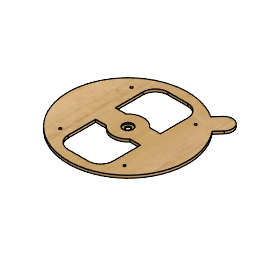
LB1-LB9 - Leveling Base Subassembly (Autodesk Fusion 360 archive; units mm, degrees)
design "LB3 - Bucket Adapter"
Autodesk Fusion 360 part; units mm, degrees
sketch "Sketch1" plane through (0, 0, 0) normal (0, 0, 1) x (1, 0, 0)
  circle A0 centre (-64.5, 71.5) radius 2.25
  circle A1 centre (64.5, 71.5) radius 2.25
  circle A2 centre (-64.5, -71.5) radius 2.25
  circle A3 centre (64.5, -71.5) radius 2.25
  line L0 (20, 100) -> (-20, 100)
  line L1 (-20, -100) -> (20, -100)
  arc A4 (-20, 100) -> (-45, 75) centre (-20, 75) ccw
  arc A5 (45, 75) -> (20, 100) centre (20, 75) ccw
  arc A6 (20, -100) -> (45, -75) centre (20, -75) ccw
  arc A7 (-45, -75) -> (-20, -100) centre (-20, -75) ccw
  line L2 (45, 20) -> (-45, -20) construction
  circle A8 centre (0, 0) radius 5
  line L3 (64.5, 71.5) -> (-64.5, 71.5) construction
  line L4 (-64.5, 71.5) -> (-64.5, -71.5) construction
  line L5 (-64.5, -71.5) -> (64.5, -71.5) construction
  line L6 (64.5, -71.5) -> (64.5, 71.5) construction
  line L7 (64.5, 71.5) -> (-64.5, -71.5) construction
  line L8 (-64.5, 71.5) -> (64.5, -71.5) construction
  line L9 (45, 20) -> (23.6854, 20)
  line L10 (-23.6854, 20) -> (-45, 20)
  line L11 (-45, 75) -> (-45, 20)
  line L12 (-45, -20) -> (-45, -75)
  arc A9 (-23.6854, -20) -> (23.6854, -20) centre (0, 0) ccw
  arc A10 (23.6854, 20) -> (-23.6854, 20) centre (0, 0) ccw
  line L13 (45, -75) -> (45, -20)
  line L14 (45, 20) -> (45, 75)
  line L15 (-45, 20) -> (4.5691, -2.0307) construction
  line L16 (28.3282, -12.5903) -> (45, -20) construction
  line L17 (-45, -20) -> (-23.6854, -20)
  line L18 (23.6854, -20) -> (45, -20)
  line L19 (91.0962, 100.9826) -> (104.4615, 88.9257) construction
  line L20 (91.0962, 100.9826) -> (77.7308, 113.0394) construction
  line L21 (104.4615, 88.9257) -> (92.8349, 76.0373)
  line L22 (77.7308, 113.0394) -> (66.1042, 100.151)
  arc A11 (104.4615, 88.9257) -> (77.7308, 113.0394) centre (91.0962, 100.9826) ccw
  arc A12 (66.1042, 100.151) -> (92.8349, 76.0373) centre (0, 0) ccw
  dimension "d14" = 4.5
  dimension "d15" = 4.5
  dimension "d16" = 4.5
  dimension "d17" = 4.5
  dimension "d20" = 240
  dimension "d21" = 25
  dimension "d23" = 40
  dimension "d24" = 10
  dimension "d25" = 62
  dimension "d26" = 129
  dimension "d27" = 143
  dimension "d29" = 36
  dimension "d33" = 45
  dimension "d34" = 100
  dimension "d35" = 100
  dimension "d36" = 149.4615
  dimension "d37" = 132.054
  dimension "d38" = 213.0394
  dimension "d39" = 18.2443
  dimension "d40" = 18
  constraint horizontal L0
  constraint perpendicular L0 L11
  constraint parallel L0 L1
  constraint parallel L11 L13
  constraint tangent L0 A4
  constraint tangent A4 L11
  constraint tangent A5 L13
  constraint tangent L0 A5
  constraint equal A4 A5
  constraint tangent L1 A6
  constraint tangent A6 L13
  constraint equal A4 A6
  constraint tangent A7 L11
  constraint tangent L1 A7
  constraint equal A4 A7
  constraint horizontal L9
  constraint parallel L9 L17
  constraint coincident L2 A8.centre
  constraint coincident A8.centre L15
  constraint coincident A8.centre A9.centre
  constraint concentric A8 A12
  constraint horizontal L3
  constraint perpendicular L3 L4
  constraint parallel L3 L5
  constraint parallel L4 L6
  constraint coincident L7 A8.centre
  constraint coincident L8 A8.centre
  constraint collinear L9 L10
  constraint coincident L10.start A9
  constraint coincident L9.end A9
  constraint collinear L11 L12
  constraint coincident L16.start L15
  constraint concentric A9 A10
  constraint collinear L13 L14
  constraint coincident A8 L15.end
  constraint collinear L15 L16
  constraint coincident A9.end L17
  constraint collinear L17 L18
  constraint coincident L19.start L20.start
  constraint tangent L21 A11
  constraint tangent L22 A11
  constraint concentric A8 A9
  constraint coincident A2.centre L4.end
  constraint coincident A1.centre L3.start
  constraint coincident A3.centre L5.end
  constraint coincident A0.centre L3.end
  measures "d14" diameter of A0
  measures "d15" diameter of A1
  measures "d16" diameter of A2
  measures "d17" diameter of A3
  measures "d20" diameter of A12
  measures "d21" radius of A4
  measures "d23" distance of L10.end L2.end
  measures "d24" diameter of A8
  measures "d25" diameter of A9
  measures "d26" distance of A2.centre A3.centre
  measures "d27" distance of A0.centre A2.centre
  measures "d29" diameter of A11
  measures "d33" distance of A8.centre L11
  measures "d34" distance of A8.centre L1
  measures "d35" distance of A8.centre L0
  measures "d36" distance of L11 L19.end
  measures "d37" angle of L3 L21
  measures "d38" distance of L1 L20.end
  measures "d39" distance of L13.end L16.start
  measures "d40" distance of L7 L21
extrude "Extrude1" add sketch "Sketch1" along normal blind 5.2
sketch "Sketch4" plane through (0, 0, 5.2) normal (0, 0, 1) x (-1, 0, 0)
  circle A0 centre (-64.5, 71.5) radius 2.25
  circle A1 centre (64.5, 71.5) radius 2.25
  line L0 (-45, -20) -> (-23.6854, -20)
  arc A2 (-23.6854, -20) -> (23.6854, -20) centre (0, 0) ccw
  line L1 (23.6854, -20) -> (45, -20)
  line L2 (45, -20) -> (45, -75)
  arc A3 (20, -100) -> (45, -75) centre (20, -75) ccw
  line L3 (20, -100) -> (-20, -100)
  arc A4 (-45, -75) -> (-20, -100) centre (-20, -75) ccw
  line L4 (-45, -75) -> (-45, -20)
  circle A5 centre (64.5, -71.5) radius 2.25
  circle A6 centre (0, 0) radius 5
  line L5 (45, 75) -> (45, 20)
  line L6 (45, 20) -> (23.6854, 20)
  arc A7 (23.6854, 20) -> (-23.6854, 20) centre (0, 0) ccw
  line L7 (-23.6854, 20) -> (-45, 20)
  line L8 (-45, 20) -> (-45, 75)
  arc A8 (-20, 100) -> (-45, 75) centre (-20, 75) ccw
  line L9 (-20, 100) -> (20, 100)
  arc A9 (45, 75) -> (20, 100) centre (20, 75) ccw
  circle A10 centre (-64.5, -71.5) radius 2.25
  arc A11 (-104.4615, -88.9257) -> (-77.7308, -113.0394) centre (-91.0962, -100.9826) ccw
  line L10 (-77.7308, -113.0394) -> (-66.1042, -100.151)
  arc A12 (-66.1042, -100.151) -> (-92.8349, -76.0373) centre (0, 0) ccw
  line L11 (-92.8349, -76.0373) -> (-104.4615, -88.9257)
  circle A13 centre (0, 0) radius 10
  dimension "d30" = 20
  constraint concentric A2 A13
  measures "d30" diameter of A13
extrude "Extrude3" cut sketch "Sketch4" against normal blind 2.6 contours A13
equation "d31 = ( -5.2 / 2 ) * 1 mm"

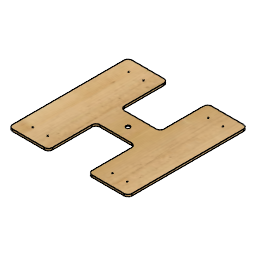
design "LB1 - Baseplate"
Autodesk Fusion 360 part; units mm, degrees
sketch "Sketch1" plane through (0, 0, 0) normal (0, 0, 1) x (1, 0, 0)
  line L0 (40, 31) -> (-40, 31)
  line L1 (-40, -31) -> (40, -31)
  line L2 (50, 31) -> (-50, -31) construction
  line L3 (-50, 31) -> (50, -31) construction
  line L4 (151, 31) -> (151, 141)
  line L5 (141, 151) -> (60, 151)
  line L6 (50, 141) -> (50, 41)
  line L7 (151, -31) -> (151, -141)
  line L8 (141, -151) -> (60, -151)
  line L9 (50, -141) -> (50, -41)
  line L10 (151, -31) -> (151, 31)
  line L11 (0, 0) -> (0, 31) construction
  line L12 (-141, 151) -> (-60, 151)
  line L13 (-50, 141) -> (-50, 41)
  line L14 (-151, 31) -> (-151, 141)
  line L15 (-151, -31) -> (-151, 31)
  line L16 (-141, -151) -> (-60, -151)
  line L17 (-50, -141) -> (-50, -41)
  line L18 (-151, -31) -> (-151, -141)
  circle A0 centre (0, 0) radius 5
  arc A1 (-141, 151) -> (-151, 141) centre (-141, 141) ccw
  arc A2 (-50, 141) -> (-60, 151) centre (-60, 141) ccw
  arc A3 (60, 151) -> (50, 141) centre (60, 141) ccw
  arc A4 (151, 141) -> (141, 151) centre (141, 141) ccw
  arc A5 (-151, -141) -> (-141, -151) centre (-141, -141) ccw
  arc A6 (-60, -151) -> (-50, -141) centre (-60, -141) ccw
  arc A7 (50, -141) -> (60, -151) centre (60, -141) ccw
  arc A8 (141, -151) -> (151, -141) centre (141, -141) ccw
  arc A9 (-40, -31) -> (-50, -41) centre (-40, -41) ccw
  arc A10 (50, -41) -> (40, -31) centre (40, -41) ccw
  arc A11 (40, 31) -> (50, 41) centre (40, 41) ccw
  arc A12 (-50, 41) -> (-40, 31) centre (-40, 41) ccw
  line L19 (100.5, -151) -> (100.5, -121) construction
  line L20 (119.25, -121) -> (81.75, -121) construction
  circle A13 centre (119.25, -121) radius 1.5
  circle A14 centre (81.75, -121) radius 1.5
  line L21 (151, 0) -> (100, 0) construction
  circle A15 centre (81.75, 121) radius 1.5
  circle A16 centre (119.25, 121) radius 1.5
  line L22 (0, -150) -> (0, -125) construction
  circle A17 centre (-81.75, -121) radius 1.5
  circle A18 centre (-119.25, -121) radius 1.5
  circle A19 centre (-81.75, 121) radius 1.5
  circle A20 centre (-119.25, 121) radius 1.5
  point P0 (50, 151)
  point P1 (50, -151)
  dimension "d1" = 100
  dimension "d2" = 62
  dimension "d3" = 101
  dimension "d4" = 120
  dimension "d5" = 101
  dimension "d6" = 120
  dimension "d9" = 10
  dimension "d10" = 10
  dimension "d11" = 30
  dimension "d12" = 18.75
  dimension "d13" = 37.5
  dimension "d14" = 3
  dimension "d15" = 3
  dimension "d21" = 51
  dimension "d22" = 25
  dimension "d23" = 125
  constraint horizontal L0
  constraint parallel L0 L1
  constraint coincident L2 L11.start
  constraint coincident L3 L11.start
  constraint coincident L11.start A0.centre
  constraint vertical L4
  constraint horizontal L5
  constraint vertical L6
  constraint vertical L7
  constraint horizontal L8
  constraint vertical L9
  constraint symmetric L4.start L11 L14.start
  constraint symmetric L7.start L11 L15.start
  constraint tangent L12 A1
  constraint tangent L14 A1
  constraint tangent L12 A2
  constraint tangent L13 A2
  constraint equal A1 A2
  constraint coincident P0 L5
  constraint coincident P0 L6
  constraint tangent L5 A3
  constraint tangent L6 A3
  constraint equal A1 A3
  constraint tangent L4 A4
  constraint tangent L5 A4
  constraint equal A1 A4
  constraint tangent L16 A5
  constraint tangent L18 A5
  constraint equal A1 A5
  constraint tangent L16 A6
  constraint tangent L17 A6
  constraint equal A1 A6
  constraint coincident P1 L8
  constraint coincident P1 L9
  constraint tangent L8 A7
  constraint tangent L9 A7
  constraint equal A1 A7
  constraint tangent L7 A8
  constraint tangent L8 A8
  constraint equal A1 A8
  constraint coincident L2.end L1
  constraint tangent L1 A9
  constraint tangent L17 A9
  constraint equal A1 A9
  constraint coincident L3.end L1
  constraint coincident L3.end L9
  constraint tangent L1 A10
  constraint tangent L9 A10
  constraint equal A1 A10
  constraint coincident L0 L11.end
  constraint coincident L2.start L6
  constraint coincident L2.start L0
  constraint tangent L6 A11
  constraint tangent L0 A11
  constraint equal A1 A11
  constraint coincident L3.start L0
  constraint tangent L13 A12
  constraint tangent L0 A12
  constraint equal A1 A12
  constraint midpoint L8 L19.start
  constraint perpendicular L8 L19
  constraint coincident L20.start A13.centre
  constraint coincident L20.end A14.centre
  constraint midpoint L10 L21.start
  constraint perpendicular L10 L21
  constraint symmetric A13 L21 A16
  constraint symmetric A14 L21 A15
  constraint vertical L22
  constraint symmetric A13 L22 A18
  constraint symmetric A14 L22 A17
  constraint symmetric A15 L22 A19
  constraint symmetric A16 L22 A20
  constraint parallel L14 L18
  constraint parallel L4 L17
  constraint parallel L1 L12
  constraint parallel L7 L14
  constraint parallel L4 L10
  constraint parallel L4 L13
  constraint parallel L4 L15
  constraint parallel L5 L16
  constraint collinear L5 L12
  constraint collinear L6 L9
  constraint collinear L8 L16
  constraint collinear L11 L22
  constraint collinear L13 L17
  constraint horizontal L20
  constraint vertical L2.end L17.start
  constraint vertical L3.start L17.start
  constraint horizontal L2.start L4.start
  constraint horizontal L19.end A18.centre
  constraint horizontal L11.start L21.end
  measures "d1" distance of L2.end L3.end
  measures "d2" distance of L3.start L2.end
  measures "d3" distance of L2.start L4.start
  measures "d4" distance of L2.start P0
  measures "d5" distance of L3.end L7.start
  measures "d6" distance of L3.end P1
  measures "d9" diameter of A0
  measures "d10" radius of A1
  measures "d11" distance of L19.start L19.end
  measures "d12" distance of L19.end L20.start
  measures "d13" distance of L20.start L20.end
  measures "d14" diameter of A13
  measures "d15" diameter of A14
  measures "d21" distance of L4 L21.end
  measures "d22" vertical distance of L22.start L22.end
  measures "d23" vertical distance of L11.start L22.end
extrude "Extrude1" add sketch "Sketch1" along normal blind 30.6
chamfer "Chamfer1" distance 5.2024 angle 41 1 edges at (-4.6616, 1.8081, 0) measured on face at (4.9938, -0.2492, 20.4)
extrude "Extrude2" cut 1 faces at (-96.5316, 12.7276, 30.6) along direction (0, 0, -1) blind 25.4
equation "d7 = 5.2 mm + 1 in"
equation "d12 = ( 37.5 / 2 ) * 1 mm"

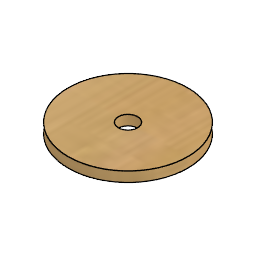
design "LB2 - Buffer Disk"
Autodesk Fusion 360 part; units mm, degrees
sketch "Sketch1" plane through (0, 0, 0) normal (0, 0, 1) x (1, 0, 0)
  circle A0 centre (0, 0) radius 31
  circle A1 centre (0, 0) radius 5
  dimension "d1" = 62
  dimension "d2" = 10
  constraint coincident A0.centre A1.centre
  constraint concentric A0 A1
  measures "d1" diameter of A0
  measures "d2" diameter of A1
extrude "Extrude1" add sketch "Sketch1" along normal blind 5.2

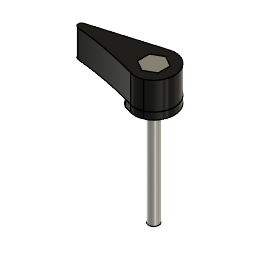
design "Lever (LB6)"
Autodesk Fusion 360 part; units mm, degrees
sketch "Sketch1" plane through (0, 0, 0) normal (0, 0, 1) x (1, 0, 0)
  circle A0 centre (0, 0) radius 1.5
  dimension "d1" = 3
  constraint coincident A0.centre origin
  measures "d1" diameter of A0
extrude "Extrude1" add sketch "Sketch1" along normal blind 28 makes body 1
sketch "Sketch2" plane through (0, 0, 28) normal (0, 0, 1) x (-1, 0, 0)
  circle A0 centre (0, 0) radius 1.5
  circle A1 centre (0, 0) radius 3
  dimension "d4" = 6
  constraint coincident A0.centre A1.centre
  measures "d4" diameter of A1
extrude "Extrude2" add sketch "Sketch2" along normal blind 2 contours A0 | A1 bodies 1
sketch "Sketch3" plane through (0, 0, 30) normal (0, 0, 1) x (-1, 0, 0)
  circle A0 centre (0, 0) radius 3
  line L0 (0, -3.5) -> (3.0311, -1.75)
  line L1 (3.0311, -1.75) -> (3.0311, 1.75)
  line L2 (3.0311, 1.75) -> (0, 3.5)
  line L3 (0, 3.5) -> (-3.0311, 1.75)
  line L4 (-3.0311, 1.75) -> (-3.0311, -1.75)
  line L5 (-3.0311, -1.75) -> (0, -3.5)
  dimension "d7" = 3.5
  constraint coincident A0.centre origin
  constraint vertical L4
  measures "d7" distance of L0.start A0.centre
extrude "Extrude3" add sketch "Sketch3" along normal blind 10 contours A0 | L0 L1 L2 L3 L4 L5 bodies 1
sketch "Sketch4" plane through (0, 0, 40) normal (0, 0, 1) x (-1, 0, 0)
  line L0 (-3.0311, -1.75) -> (0, -3.5)
  line L1 (0, -3.5) -> (3.0311, -1.75)
  line L2 (3.0311, -1.75) -> (3.0311, 1.75)
  line L3 (3.0311, 1.75) -> (0, 3.5)
  line L4 (0, 3.5) -> (-3.0311, 1.75)
  line L5 (-3.0311, 1.75) -> (-3.0311, -1.75)
  line L6 (1.0405, -5.7108) -> (20.2864, 0.0419)
  arc A0 (0.9798, 5.7098) -> (20.1005, 1.9949) centre (30.843, 108.3515) ccw
  arc A1 (20.2864, 0.0419) -> (20.1005, 1.9949) centre (20, 1) ccw
  arc A2 (-2.502, 5.4535) -> (-2.3485, -5.5213) centre (0, 0) ccw
  arc A3 (-2.3485, -5.5213) -> (1.0405, -5.7108) centre (-0.3914, -0.9202) ccw
  arc A4 (0.9798, 5.7098) -> (-2.502, 5.4535) centre (-0.417, 0.9089) ccw
  dimension "d10" = 12
  dimension "d12" = 1
  dimension "d13" = 20
  dimension "d14" = 5
  dimension "d20" = 5
  dimension "d21" = 106.8978
  dimension "d22" = 0.8298
  dimension "d23" = 2.6141
  dimension "d24" = 33.8741
  constraint coincident A2.centre origin
  constraint tangent L6 A1
  constraint tangent A0 A1
  constraint tangent L6 A3
  constraint tangent A2 A3
  constraint tangent A0 A4
  constraint tangent A2 A4
  measures "d10" diameter of A2
  measures "d12" radius of A1
  measures "d13" horizontal distance of A2.centre A1.centre
  measures "d14" radius of A3
  measures "d20" radius of A4
  measures "d21" radius of A0
  measures "d22" vertical distance of L0.start A3.centre
  measures "d23" distance of L5 A4.centre
  measures "d24" distance of L5 A0.centre
extrude "Extrude4" add sketch "Sketch4" against normal blind 8 separate body makes body 2
sketch "Sketch5" plane through (0, 0, 32) normal (0, 0, -1) x (1, 0, 0)
  line L0 (3.0311, 1.75) -> (3.0311, -1.75)
  line L1 (3.0311, -1.75) -> (0, -3.5)
  line L2 (0, -3.5) -> (-3.0311, -1.75)
  line L3 (-3.0311, -1.75) -> (-3.0311, 1.75)
  line L4 (-3.0311, 1.75) -> (0, 3.5)
  line L5 (0, 3.5) -> (3.0311, 1.75)
  arc A0 (2.3485, -5.5213) -> (2.502, 5.4535) centre (0, 0) ccw
  arc A1 (-20.1005, 1.9949) -> (-0.9798, 5.7098) centre (-30.843, 108.3515) ccw
  arc A2 (-20.1005, 1.9949) -> (-20.2864, 0.0419) centre (-20, 1) ccw
  line L6 (-20.2864, 0.0419) -> (-1.0405, -5.7108)
  arc A3 (-1.0405, -5.7108) -> (2.3485, -5.5213) centre (0.3914, -0.9202) ccw
  circle A4 centre (0, 0) radius 6
  arc A5 (2.502, 5.4535) -> (-0.9798, 5.7098) centre (0.417, 0.9089) ccw
  dimension "d17" = 12
  constraint coincident A0.centre A4.centre
  measures "d17" diameter of A4
extrude "Extrude5" add sketch "Sketch5" along normal blind 2 separate body contours A0 A1 L6 A3 A4 A5 makes body 3
equation "d2 = ( 55 / 2 ) * 1 mm + 0.5 mm"
